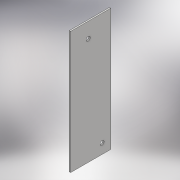
# Autodesk Inventor part: stay
Saved by Autodesk Inventor 2018.2 (Build 222227000, 227)
## iProperties
Created: 2017-12-11
Part Number: stay
Material: 一般
Document SubType Name: Modeling
Designer: kuwano
Density: 1 g/cm^3
Appearance: 既定
Author: kuwano
Autodesk Inventor part; units mm, degrees
ref_plane "YZ Plane" through (0, 0, 0) normal (1, 0, 0) x (0, 1, 0)
ref_plane "XZ Plane" through (0, 0, 0) normal (0, 1, 0) x (-1, 0, 0)
ref_plane "XY Plane" through (0, 0, 0) normal (0, 0, 1) x (1, 0, 0)
sketch "スケッチ1" plane through (0, 0, 0) normal (1, 0, 0) x (0, 1, 0)
  circle A0 centre (0, 0) radius 7.5
  circle A1 centre (50, -350) radius 7.5
  line L0 (81.3202, 54.372) -> (-63.1061, 54.372)
  line L1 (-63.1061, 54.372) -> (-63.1061, -385.952)
  line L2 (-63.1061, -385.952) -> (81.3202, -385.952)
  line L3 (81.3202, -385.952) -> (81.3202, 54.372)
  dimension "d0" = 50
  dimension "d1" = 350
  dimension "d2" = 15
  dimension "d3" = 15
  constraints: 8 end point, 2 centre point, 2 parallel, 1 coincident, 1 horizontal, 1 perpendicular
  measures "d0" horizontal distance of A1.centre A0.centre
  measures "d1" vertical distance of A0.centre A1.centre
  measures "d2" diameter of A0
  measures "d3" diameter of A1
extrude "押し出し1" add sketch "スケッチ1" along normal mid plane 5
